Autodesk Fusion 360 part; units mm, degrees
note: some values were not read from the file. Set by a fixed rule: which face or edge a step refers to.
(part 3 of 3)
sketch "Sketch13" plane through (0, 0, 5) normal (0, 0, 1) x (-1, 0, 0)
  line L0 (7, 166) -> (25, 166)
  line L1 (25, 166) -> (25, 167)
  line L2 (25, 167) -> (-35, 167)
  line L3 (-35, 167) -> (-35, 166)
  line L4 (-35, 166) -> (-17, 166)
  line L5 (-17, 166) -> (-17, 164)
  line L6 (-17, 164) -> (-35, 164)
  line L7 (-35, 164) -> (-35, 156)
  line L8 (-35, 156) -> (-17, 156)
  line L9 (-17, 156) -> (-17, 154)
  line L10 (-17, 154) -> (-35, 154)
  line L11 (-35, 154) -> (-35, 146)
  line L12 (-35, 146) -> (-17, 146)
  line L13 (-17, 146) -> (-17, 144)
  line L14 (-17, 144) -> (-35, 144)
  line L15 (-35, 144) -> (-35, 138)
  line L16 (-35, 138) -> (-17, 138)
  line L17 (-17, 138) -> (-17, 136)
  line L18 (-17, 136) -> (-35, 136)
  line L19 (-35, 136) -> (-35, 130)
  line L20 (-35, 130) -> (-17, 130)
  line L21 (-17, 130) -> (-17, 128)
  line L22 (-17, 128) -> (-35, 128)
  line L23 (-35, 128) -> (-35, 122)
  line L24 (-35, 122) -> (-17, 122)
  line L25 (-17, 122) -> (-17, 120)
  line L26 (-17, 120) -> (-35, 120)
  line L27 (-35, 120) -> (-35, 114)
  line L28 (-35, 114) -> (-17, 114)
  line L29 (-17, 114) -> (-17, 112)
  line L30 (-17, 112) -> (-35, 112)
  line L31 (-35, 112) -> (-35, 106)
  line L32 (-35, 106) -> (-17, 106)
  line L33 (-17, 106) -> (-17, 104)
  line L34 (-17, 104) -> (-35, 104)
  line L35 (-35, 104) -> (-35, 98)
  line L36 (-35, 98) -> (-17, 98)
  line L37 (-17, 98) -> (-17, 96)
  line L38 (-17, 96) -> (-35, 96)
  line L39 (-35, 96) -> (-35, 90)
  line L40 (-35, 90) -> (-17, 90)
  line L41 (-17, 90) -> (-17, 88)
  line L42 (-17, 88) -> (-35, 88)
  line L43 (-35, 88) -> (-35, 82)
  line L44 (-35, 82) -> (-17, 82)
  line L45 (-17, 82) -> (-17, 80)
  line L46 (-17, 80) -> (-35, 80)
  line L47 (-35, 80) -> (-35, 74)
  line L48 (-35, 74) -> (-17, 74)
  line L49 (-17, 74) -> (-17, 72)
  line L50 (-17, 72) -> (-35, 72)
  line L51 (-35, 72) -> (-35, 66)
  line L52 (-35, 66) -> (-17, 66)
  line L53 (-17, 66) -> (-17, 64)
  line L54 (-17, 64) -> (-35, 64)
  line L55 (-35, 64) -> (-35, 58)
  line L56 (-35, 58) -> (-17, 58)
  line L57 (-17, 58) -> (-17, 56)
  line L58 (-17, 56) -> (-35, 56)
  line L59 (-35, 56) -> (-35, 50)
  line L60 (-35, 50) -> (-17, 50)
  line L61 (-17, 50) -> (-17, 48)
  line L62 (-17, 48) -> (-35, 48)
  line L63 (-35, 48) -> (-35, 42)
  line L64 (-35, 42) -> (-17, 42)
  line L65 (-17, 42) -> (-17, 40)
  line L66 (-17, 40) -> (-35, 40)
  line L67 (-35, 40) -> (-35, 34)
  line L68 (-35, 34) -> (-17, 34)
  line L69 (-17, 34) -> (-17, 32)
  line L70 (-17, 32) -> (-35, 32)
  line L71 (-35, 32) -> (-35, 26)
  line L72 (-35, 26) -> (-17, 26)
  line L73 (-17, 26) -> (-17, 24)
  line L74 (-17, 24) -> (-35, 24)
  line L75 (-35, 24) -> (-35, 18)
  line L76 (-35, 18) -> (-17, 18)
  line L77 (-17, 18) -> (-17, 16)
  line L78 (-17, 16) -> (-35, 16)
  line L79 (-35, 16) -> (-35, 10)
  line L80 (-35, 10) -> (-17, 10)
  line L81 (-17, 10) -> (-17, 8)
  line L82 (-17, 8) -> (-35, 8)
  line L83 (-35, 8) -> (-35, 2)
  line L84 (-35, 2) -> (-17, 2)
  line L85 (-17, 2) -> (-17, 0)
  line L86 (-17, 0) -> (-35, 0)
  line L87 (-35, 0) -> (-35, -6)
  line L88 (-35, -6) -> (-17, -6)
  line L89 (-17, -6) -> (-17, -8)
  line L90 (-17, -8) -> (-35, -8)
  line L91 (-35, -8) -> (-35, -14)
  line L92 (-35, -14) -> (-17, -14)
  line L93 (-17, -14) -> (-17, -16)
  line L94 (-17, -16) -> (-35, -16)
  line L95 (-35, -16) -> (-35, -22)
  line L96 (-35, -22) -> (-17, -22)
  line L97 (-17, -22) -> (-17, -24)
  line L98 (-17, -24) -> (-35, -24)
  line L99 (-35, -24) -> (-35, -32)
  line L100 (-35, -32) -> (-17, -32)
  line L101 (-17, -32) -> (-17, -34)
  line L102 (-17, -34) -> (-35, -34)
  line L103 (-35, -34) -> (-35, -42)
  line L104 (-35, -42) -> (-40, -42)
  line L105 (-40, -42) -> (-40, -70)
  line L106 (-40, -70) -> (30, -70)
  line L107 (30, -70) -> (30, -42)
  line L108 (30, -42) -> (25, -42)
  line L109 (25, -42) -> (25, -34)
  line L110 (25, -34) -> (7, -34)
  line L111 (7, -34) -> (7, -32)
  line L112 (7, -32) -> (25, -32)
  line L113 (25, -32) -> (25, -24)
  line L114 (25, -24) -> (7, -24)
  line L115 (7, -24) -> (7, -22)
  line L116 (7, -22) -> (25, -22)
  line L117 (25, -22) -> (25, -16)
  line L118 (25, -16) -> (7, -16)
  line L119 (7, -16) -> (7, -14)
  line L120 (7, -14) -> (25, -14)
  line L121 (25, -14) -> (25, -8)
  line L122 (25, -8) -> (7, -8)
  line L123 (7, -8) -> (7, -6)
  line L124 (7, -6) -> (25, -6)
  line L125 (25, -6) -> (25, 0)
  line L126 (25, 0) -> (7, 0)
  line L127 (7, 0) -> (7, 2)
  line L128 (7, 2) -> (25, 2)
  line L129 (25, 2) -> (25, 8)
  line L130 (25, 8) -> (7, 8)
  line L131 (7, 8) -> (7, 10)
  line L132 (7, 10) -> (25, 10)
  line L133 (25, 10) -> (25, 16)
  line L134 (25, 16) -> (7, 16)
  line L135 (7, 16) -> (7, 18)
  line L136 (7, 18) -> (25, 18)
  line L137 (25, 18) -> (25, 24)
  line L138 (25, 24) -> (7, 24)
  line L139 (7, 24) -> (7, 26)
  line L140 (7, 26) -> (25, 26)
  line L141 (25, 26) -> (25, 32)
  line L142 (25, 32) -> (7, 32)
  line L143 (7, 32) -> (7, 34)
  line L144 (7, 34) -> (25, 34)
  line L145 (25, 34) -> (25, 40)
  line L146 (25, 40) -> (7, 40)
  line L147 (7, 40) -> (7, 42)
  line L148 (7, 42) -> (25, 42)
  line L149 (25, 42) -> (25, 48)
  line L150 (25, 48) -> (7, 48)
  line L151 (7, 48) -> (7, 50)
  line L152 (7, 50) -> (25, 50)
  line L153 (25, 50) -> (25, 56)
  line L154 (25, 56) -> (7, 56)
  line L155 (7, 56) -> (7, 58)
  line L156 (7, 58) -> (25, 58)
  line L157 (25, 58) -> (25, 64)
  line L158 (25, 64) -> (7, 64)
  line L159 (7, 64) -> (7, 66)
  line L160 (7, 66) -> (25, 66)
  line L161 (25, 66) -> (25, 72)
  line L162 (25, 72) -> (7, 72)
  line L163 (7, 72) -> (7, 74)
  line L164 (7, 74) -> (25, 74)
  line L165 (25, 74) -> (25, 80)
  line L166 (25, 80) -> (7, 80)
  line L167 (7, 80) -> (7, 82)
  line L168 (7, 82) -> (25, 82)
  line L169 (25, 82) -> (25, 88)
  line L170 (25, 88) -> (7, 88)
  line L171 (7, 88) -> (7, 90)
  line L172 (7, 90) -> (25, 90)
  line L173 (25, 90) -> (25, 96)
  line L174 (25, 96) -> (7, 96)
  line L175 (7, 96) -> (7, 98)
  line L176 (7, 98) -> (25, 98)
  line L177 (25, 98) -> (25, 104)
  line L178 (25, 104) -> (7, 104)
  line L179 (7, 104) -> (7, 106)
  line L180 (7, 106) -> (25, 106)
  line L181 (25, 106) -> (25, 112)
  line L182 (25, 112) -> (7, 112)
  line L183 (7, 112) -> (7, 114)
  line L184 (7, 114) -> (25, 114)
  line L185 (25, 114) -> (25, 120)
  line L186 (25, 120) -> (7, 120)
  line L187 (7, 120) -> (7, 122)
  line L188 (7, 122) -> (25, 122)
  line L189 (25, 122) -> (25, 128)
  line L190 (25, 128) -> (7, 128)
  line L191 (7, 128) -> (7, 130)
  line L192 (7, 130) -> (25, 130)
  line L193 (25, 130) -> (25, 136)
  line L194 (25, 136) -> (7, 136)
  line L195 (7, 136) -> (7, 138)
  line L196 (7, 138) -> (25, 138)
  line L197 (25, 138) -> (25, 144)
  line L198 (25, 144) -> (7, 144)
  line L199 (7, 144) -> (7, 146)
  line L200 (7, 146) -> (25, 146)
  line L201 (25, 146) -> (25, 154)
  line L202 (25, 154) -> (7, 154)
  line L203 (7, 154) -> (7, 156)
  line L204 (7, 156) -> (25, 156)
  line L205 (25, 156) -> (25, 164)
  line L206 (25, 164) -> (7, 164)
  line L207 (7, 164) -> (7, 166)
  line L208 (23, -29) -> (-33, -29)
  line L209 (-33, -29) -> (-33, -27)
  line L210 (-33, -27) -> (23, -27)
  line L211 (23, -27) -> (23, -29)
  line L212 (4, -32) -> (4, -34)
  line L213 (4, -34) -> (-14, -34)
  line L214 (-14, -34) -> (-14, -32)
  line L215 (-14, -32) -> (4, -32)
  line L216 (23, -39) -> (-33, -39)
  line L217 (-33, -39) -> (-33, -37)
  line L218 (-33, -37) -> (23, -37)
  line L219 (23, -37) -> (23, -39)
  line L220 (4, 146) -> (4, 144)
  line L221 (4, 144) -> (-14, 144)
  line L222 (-14, 144) -> (-14, 146)
  line L223 (-14, 146) -> (4, 146)
  line L224 (23, 78) -> (23, 76)
  line L225 (23, 76) -> (-33, 76)
  line L226 (-33, 76) -> (-33, 78)
  line L227 (-33, 78) -> (23, 78)
  line L228 (-33, 94) -> (23, 94)
  line L229 (23, 94) -> (23, 92)
  line L230 (23, 92) -> (-33, 92)
  line L231 (-33, 92) -> (-33, 94)
  line L232 (23, 54) -> (23, 52)
  line L233 (23, 52) -> (-33, 52)
  line L234 (-33, 52) -> (-33, 54)
  line L235 (-33, 54) -> (23, 54)
  line L236 (4, 66) -> (4, 64)
  line L237 (4, 64) -> (-14, 64)
  line L238 (-14, 64) -> (-14, 66)
  line L239 (-14, 66) -> (4, 66)
  line L240 (4, 106) -> (4, 104)
  line L241 (4, 104) -> (-14, 104)
  line L242 (-14, 104) -> (-14, 106)
  line L243 (-14, 106) -> (4, 106)
  line L244 (23, 102) -> (23, 100)
  line L245 (23, 100) -> (-32.9874, 100)
  line L246 (-32.9874, 100) -> (-32.9874, 102)
  line L247 (-32.9874, 102) -> (23, 102)
  line L248 (4, 50) -> (4, 48)
  line L249 (4, 48) -> (-14, 48)
  line L250 (-14, 48) -> (-14, 50)
  line L251 (-14, 50) -> (4, 50)
  line L252 (4, 90) -> (4, 88)
  line L253 (4, 88) -> (-14, 88)
  line L254 (-14, 88) -> (-14, 90)
  line L255 (-14, 90) -> (4, 90)
  line L256 (4, 74) -> (4, 72)
  line L257 (4, 72) -> (-14, 72)
  line L258 (-14, 72) -> (-14, 74)
  line L259 (-14, 74) -> (4, 74)
  line L260 (23, 62) -> (23, 60)
  line L261 (23, 60) -> (-33, 60)
  line L262 (-33, 60) -> (-33, 62)
  line L263 (-33, 62) -> (23, 62)
  line L264 (-33, 116) -> (-33, 118)
  line L265 (-33, 118) -> (23, 118)
  line L266 (23, 118) -> (23, 116)
  line L267 (23, 116) -> (-33, 116)
  line L268 (4, 82) -> (4, 80)
  line L269 (4, 80) -> (-14, 80)
  line L270 (-14, 80) -> (-14, 82)
  line L271 (-14, 82) -> (4, 82)
  line L272 (4, 42) -> (4, 40)
  line L273 (4, 40) -> (-14, 40)
  line L274 (-14, 40) -> (-14, 42)
  line L275 (-14, 42) -> (4, 42)
  line L276 (23, 70) -> (23, 68)
  line L277 (23, 68) -> (-33, 68)
  line L278 (-33, 68) -> (-33, 70)
  line L279 (-33, 70) -> (23, 70)
  line L280 (23, 110) -> (23, 108)
  line L281 (23, 108) -> (-33, 108)
  line L282 (-33, 108) -> (-33, 110)
  line L283 (-33, 110) -> (23, 110)
  line L284 (4, 114) -> (4, 112)
  line L285 (4, 112) -> (-14, 112)
  line L286 (-14, 112) -> (-14, 114)
  line L287 (-14, 114) -> (4, 114)
  line L288 (4, 98) -> (4, 96)
  line L289 (4, 96) -> (-14, 96)
  line L290 (-14, 96) -> (-14, 98)
  line L291 (-14, 98) -> (4, 98)
  line L292 (23, 46.2715) -> (23, 44)
  line L293 (23, 44) -> (-33, 44)
  line L294 (-33, 44) -> (-33, 46.2715)
  line L295 (-33, 46.2715) -> (23, 46.2715)
  line L296 (23, 86) -> (23, 84)
  line L297 (23, 84) -> (-33, 84)
  line L298 (-33, 84) -> (-33, 86)
  line L299 (-33, 86) -> (23, 86)
  line L300 (4, 58) -> (4, 56)
  line L301 (4, 56) -> (-14, 56)
  line L302 (-14, 56) -> (-14, 58)
  line L303 (-14, 58) -> (4, 58)
  line L304 (23, -18) -> (23, -20)
  line L305 (23, -20) -> (-33, -20)
  line L306 (-33, -20) -> (-33, -18)
  line L307 (-33, -18) -> (23, -18)
  line L308 (4, -24) -> (-14, -24)
  line L309 (-14, -24) -> (-14, -22)
  line L310 (-14, -22) -> (4, -22)
  line L311 (4, -22) -> (4, -24)
  line L312 (23, 22) -> (23, 20)
  line L313 (23, 20) -> (-33, 20)
  line L314 (-33, 20) -> (-33, 22)
  line L315 (-33, 22) -> (23, 22)
  line L316 (23, 6) -> (23, 4)
  line L317 (23, 4) -> (-33, 4)
  line L318 (-33, 4) -> (-33, 6)
  line L319 (-33, 6) -> (23, 6)
  line L320 (23, -10) -> (23, -12)
  line L321 (23, -12) -> (-33, -12)
  line L322 (-33, -12) -> (-33, -10)
  line L323 (-33, -10) -> (23, -10)
  line L324 (4, -14) -> (4, -16)
  line L325 (4, -16) -> (-14, -16)
  line L326 (-14, -16) -> (-14, -14)
  line L327 (-14, -14) -> (4, -14)
  line L328 (4, -6) -> (4, -8)
  line L329 (4, -8) -> (-14, -8)
  line L330 (-14, -8) -> (-14, -6)
  line L331 (-14, -6) -> (4, -6)
  line L332 (4, 10) -> (4, 8)
  line L333 (4, 8) -> (-14, 8)
  line L334 (-14, 8) -> (-14, 10)
  line L335 (-14, 10) -> (4, 10)
  line L336 (4, 26) -> (4, 24)
  line L337 (4, 24) -> (-14, 24)
  line L338 (-14, 24) -> (-14, 26)
  line L339 (-14, 26) -> (4, 26)
  line L340 (4, 34) -> (4, 32)
  line L341 (4, 32) -> (-14, 32)
  line L342 (-14, 32) -> (-14, 34)
  line L343 (-14, 34) -> (4, 34)
  line L344 (4, 18) -> (4, 16)
  line L345 (4, 16) -> (-14, 16)
  line L346 (-14, 16) -> (-14, 18)
  line L347 (-14, 18) -> (4, 18)
  line L348 (4, 2) -> (4, 0)
  line L349 (4, 0) -> (-14, 0)
  line L350 (-14, 0) -> (-14, 2)
  line L351 (-14, 2) -> (4, 2)
  line L352 (23, 38) -> (23, 36)
  line L353 (23, 36) -> (-33, 36)
  line L354 (-33, 36) -> (-33, 38)
  line L355 (-33, 38) -> (23, 38)
  line L356 (23, -2) -> (23, -4)
  line L357 (23, -4) -> (-33, -4)
  line L358 (-33, -4) -> (-33, -2)
  line L359 (-33, -2) -> (23, -2)
  line L360 (23, 14) -> (23, 12)
  line L361 (23, 12) -> (-33, 12)
  line L362 (-33, 12) -> (-33, 14)
  line L363 (-33, 14) -> (23, 14)
  line L364 (23, 30) -> (23, 28)
  line L365 (23, 28) -> (-33, 28)
  line L366 (-33, 28) -> (-33, 30)
  line L367 (-33, 30) -> (23, 30)
  line L368 (4, 122) -> (4, 120)
  line L369 (4, 120) -> (-14, 120)
  line L370 (-14, 120) -> (-14, 122)
  line L371 (-14, 122) -> (4, 122)
  line L372 (4, 138) -> (4, 136)
  line L373 (4, 136) -> (-14, 136)
  line L374 (-14, 136) -> (-14, 138)
  line L375 (-14, 138) -> (4, 138)
  line L376 (4, 130) -> (4, 128)
  line L377 (4, 128) -> (-14, 128)
  line L378 (-14, 128) -> (-14, 130)
  line L379 (-14, 130) -> (4, 130)
  line L380 (23, 126) -> (23, 124)
  line L381 (23, 124) -> (-33, 124)
  line L382 (-33, 124) -> (-33, 126)
  line L383 (-33, 126) -> (23, 126)
  line L384 (23, 142) -> (23, 140)
  line L385 (23, 140) -> (-33, 140)
  line L386 (-33, 140) -> (-33, 142)
  line L387 (-33, 142) -> (23, 142)
  line L388 (23, 134) -> (23, 132)
  line L389 (23, 132) -> (-33, 132)
  line L390 (-33, 132) -> (-33, 134)
  line L391 (-33, 134) -> (23, 134)
  line L392 (23, 151) -> (23, 149)
  line L393 (23, 149) -> (-33, 149)
  line L394 (-33, 149) -> (-33, 151)
  line L395 (-33, 151) -> (23, 151)
  line L396 (4, 156) -> (4, 154)
  line L397 (4, 154) -> (-14, 154)
  line L398 (-14, 154) -> (-14, 156)
  line L399 (-14, 156) -> (4, 156)
  line L400 (23, 161) -> (23, 159)
  line L401 (23, 159) -> (-33, 159)
  line L402 (-33, 159) -> (-33, 161)
  line L403 (-33, 161) -> (23, 161)
  line L404 (-14, 164) -> (-14, 166)
  line L405 (-14, 166) -> (4, 166)
  line L406 (4, 166) -> (4, 164)
  line L407 (4, 164) -> (-14, 164)
  line L408 (30, -42) -> (-40, -42)
  line L409 (-40, -42) -> (-40, -70)
  line L410 (-40, -70) -> (30, -70)
  line L411 (30, -70) -> (30, -42)
  constraint horizontal L408
  constraint vertical L409
  constraint horizontal L410
  constraint vertical L411
  constraint coincident L105.end L106.start
  constraint coincident L107.end L108.start
extrude "Extrude20" add sketch "Sketch13" along normal blind 2.5 contours L104 L105 L106 L107 L108 L408 L409 L410 L411
sketch "Sketch14" plane through (0, 0, 0) normal (0, 0, -1) x (1, 0, 0)
  line L0 (-25, 166) -> (-7, 166)
  line L1 (-7, 166) -> (-7, 164)
  line L2 (-7, 164) -> (-25, 164)
  line L3 (-25, 164) -> (-25, 156)
  line L4 (-25, 156) -> (-7, 156)
  line L5 (-7, 156) -> (-7, 154)
  line L6 (-7, 154) -> (-25, 154)
  line L7 (-25, 154) -> (-25, 146)
  line L8 (-25, 146) -> (-7, 146)
  line L9 (-7, 146) -> (-7, 144)
  line L10 (-7, 144) -> (-25, 144)
  line L11 (-25, 144) -> (-25, 138)
  line L12 (-25, 138) -> (-7, 138)
  line L13 (-7, 138) -> (-7, 136)
  line L14 (-7, 136) -> (-25, 136)
  line L15 (-25, 136) -> (-25, 130)
  line L16 (-25, 130) -> (-7, 130)
  line L17 (-7, 130) -> (-7, 128)
  line L18 (-7, 128) -> (-25, 128)
  line L19 (-25, 128) -> (-25, 122)
  line L20 (-25, 122) -> (-7, 122)
  line L21 (-7, 122) -> (-7, 120)
  line L22 (-7, 120) -> (-25, 120)
  line L23 (-25, 120) -> (-25, 114)
  line L24 (-25, 114) -> (-7, 114)
  line L25 (-7, 114) -> (-7, 112)
  line L26 (-7, 112) -> (-25, 112)
  line L27 (-25, 112) -> (-25, 106)
  line L28 (-25, 106) -> (-7, 106)
  line L29 (-7, 106) -> (-7, 104)
  line L30 (-7, 104) -> (-25, 104)
  line L31 (-25, 104) -> (-25, 98)
  line L32 (-25, 98) -> (-7, 98)
  line L33 (-7, 98) -> (-7, 96)
  line L34 (-7, 96) -> (-25, 96)
  line L35 (-25, 96) -> (-25, 90)
  line L36 (-25, 90) -> (-7, 90)
  line L37 (-7, 90) -> (-7, 88)
  line L38 (-7, 88) -> (-25, 88)
  line L39 (-25, 88) -> (-25, 82)
  line L40 (-25, 82) -> (-7, 82)
  line L41 (-7, 82) -> (-7, 80)
  line L42 (-7, 80) -> (-25, 80)
  line L43 (-25, 80) -> (-25, 74)
  line L44 (-25, 74) -> (-7, 74)
  line L45 (-7, 74) -> (-7, 72)
  line L46 (-7, 72) -> (-25, 72)
  line L47 (-25, 72) -> (-25, 66)
  line L48 (-25, 66) -> (-7, 66)
  line L49 (-7, 66) -> (-7, 64)
  line L50 (-7, 64) -> (-25, 64)
  line L51 (-25, 64) -> (-25, 58)
  line L52 (-25, 58) -> (-7, 58)
  line L53 (-7, 58) -> (-7, 56)
  line L54 (-7, 56) -> (-25, 56)
  line L55 (-25, 56) -> (-25, 50)
  line L56 (-25, 50) -> (-7, 50)
  line L57 (-7, 50) -> (-7, 48)
  line L58 (-7, 48) -> (-25, 48)
  line L59 (-25, 48) -> (-25, 42)
  line L60 (-25, 42) -> (-7, 42)
  line L61 (-7, 42) -> (-7, 40)
  line L62 (-7, 40) -> (-25, 40)
  line L63 (-25, 40) -> (-25, 34)
  line L64 (-25, 34) -> (-7, 34)
  line L65 (-7, 34) -> (-7, 32)
  line L66 (-7, 32) -> (-25, 32)
  line L67 (-25, 32) -> (-25, 26)
  line L68 (-25, 26) -> (-7, 26)
  line L69 (-7, 26) -> (-7, 24)
  line L70 (-7, 24) -> (-25, 24)
  line L71 (-25, 24) -> (-25, 18)
  line L72 (-25, 18) -> (-7, 18)
  line L73 (-7, 18) -> (-7, 16)
  line L74 (-7, 16) -> (-25, 16)
  line L75 (-25, 16) -> (-25, 10)
  line L76 (-25, 10) -> (-7, 10)
  line L77 (-7, 10) -> (-7, 8)
  line L78 (-7, 8) -> (-25, 8)
  line L79 (-25, 8) -> (-25, 2)
  line L80 (-25, 2) -> (-7, 2)
  line L81 (-7, 2) -> (-7, 0)
  line L82 (-7, 0) -> (-25, 0)
  line L83 (-25, 0) -> (-25, -6)
  line L84 (-25, -6) -> (-7, -6)
  line L85 (-7, -6) -> (-7, -8)
  line L86 (-7, -8) -> (-25, -8)
  line L87 (-25, -8) -> (-25, -14)
  line L88 (-25, -14) -> (-7, -14)
  line L89 (-7, -14) -> (-7, -16)
  line L90 (-7, -16) -> (-25, -16)
  line L91 (-25, -16) -> (-25, -22)
  line L92 (-25, -22) -> (-7, -22)
  line L93 (-7, -22) -> (-7, -24)
  line L94 (-7, -24) -> (-25, -24)
  line L95 (-25, -24) -> (-25, -32)
  line L96 (-25, -32) -> (-7, -32)
  line L97 (-7, -32) -> (-7, -34)
  line L98 (-7, -34) -> (-25, -34)
  line L99 (-25, -34) -> (-25, -42)
  line L100 (-25, -42) -> (-30, -42)
  line L101 (-30, -42) -> (-30, -70)
  line L102 (-30, -70) -> (40, -70)
  line L103 (40, -70) -> (40, -42)
  line L104 (40, -42) -> (35, -42)
  line L105 (35, -42) -> (35, -34)
  line L106 (35, -34) -> (17, -34)
  line L107 (17, -34) -> (17, -32)
  line L108 (17, -32) -> (35, -32)
  line L109 (35, -32) -> (35, -24)
  line L110 (35, -24) -> (17, -24)
  line L111 (17, -24) -> (17, -22)
  line L112 (17, -22) -> (35, -22)
  line L113 (35, -22) -> (35, -16)
  line L114 (35, -16) -> (17, -16)
  line L115 (17, -16) -> (17, -14)
  line L116 (17, -14) -> (35, -14)
  line L117 (35, -14) -> (35, -8)
  line L118 (35, -8) -> (17, -8)
  line L119 (17, -8) -> (17, -6)
  line L120 (17, -6) -> (35, -6)
  line L121 (35, -6) -> (35, 0)
  line L122 (35, 0) -> (17, 0)
  line L123 (17, 0) -> (17, 2)
  line L124 (17, 2) -> (35, 2)
  line L125 (35, 2) -> (35, 8)
  line L126 (35, 8) -> (17, 8)
  line L127 (17, 8) -> (17, 10)
  line L128 (17, 10) -> (35, 10)
  line L129 (35, 10) -> (35, 16)
  line L130 (35, 16) -> (17, 16)
  line L131 (17, 16) -> (17, 18)
  line L132 (17, 18) -> (35, 18)
  line L133 (35, 18) -> (35, 24)
  line L134 (35, 24) -> (17, 24)
  line L135 (17, 24) -> (17, 26)
  line L136 (17, 26) -> (35, 26)
  line L137 (35, 26) -> (35, 32)
  line L138 (35, 32) -> (17, 32)
  line L139 (17, 32) -> (17, 34)
  line L140 (17, 34) -> (35, 34)
  line L141 (35, 34) -> (35, 40)
  line L142 (35, 40) -> (17, 40)
  line L143 (17, 40) -> (17, 42)
  line L144 (17, 42) -> (35, 42)
  line L145 (35, 42) -> (35, 48)
  line L146 (35, 48) -> (17, 48)
  line L147 (17, 48) -> (17, 50)
  line L148 (17, 50) -> (35, 50)
  line L149 (35, 50) -> (35, 56)
  line L150 (35, 56) -> (17, 56)
  line L151 (17, 56) -> (17, 58)
  line L152 (17, 58) -> (35, 58)
  line L153 (35, 58) -> (35, 64)
  line L154 (35, 64) -> (17, 64)
  line L155 (17, 64) -> (17, 66)
  line L156 (17, 66) -> (35, 66)
  line L157 (35, 66) -> (35, 72)
  line L158 (35, 72) -> (17, 72)
  line L159 (17, 72) -> (17, 74)
  line L160 (17, 74) -> (35, 74)
  line L161 (35, 74) -> (35, 80)
  line L162 (35, 80) -> (17, 80)
  line L163 (17, 80) -> (17, 82)
  line L164 (17, 82) -> (35, 82)
  line L165 (35, 82) -> (35, 88)
  line L166 (35, 88) -> (17, 88)
  line L167 (17, 88) -> (17, 90)
  line L168 (17, 90) -> (35, 90)
  line L169 (35, 90) -> (35, 96)
  line L170 (35, 96) -> (17, 96)
  line L171 (17, 96) -> (17, 98)
  line L172 (17, 98) -> (35, 98)
  line L173 (35, 98) -> (35, 104)
  line L174 (35, 104) -> (17, 104)
  line L175 (17, 104) -> (17, 106)
  line L176 (17, 106) -> (35, 106)
  line L177 (35, 106) -> (35, 112)
  line L178 (35, 112) -> (17, 112)
  line L179 (17, 112) -> (17, 114)
  line L180 (17, 114) -> (35, 114)
  line L181 (35, 114) -> (35, 120)
  line L182 (35, 120) -> (17, 120)
  line L183 (17, 120) -> (17, 122)
  line L184 (17, 122) -> (35, 122)
  line L185 (35, 122) -> (35, 128)
  line L186 (35, 128) -> (17, 128)
  line L187 (17, 128) -> (17, 130)
  line L188 (17, 130) -> (35, 130)
  line L189 (35, 130) -> (35, 136)
  line L190 (35, 136) -> (17, 136)
  line L191 (17, 136) -> (17, 138)
  line L192 (17, 138) -> (35, 138)
  line L193 (35, 138) -> (35, 144)
  line L194 (35, 144) -> (17, 144)
  line L195 (17, 144) -> (17, 146)
  line L196 (17, 146) -> (35, 146)
  line L197 (35, 146) -> (35, 154)
  line L198 (35, 154) -> (17, 154)
  line L199 (17, 154) -> (17, 156)
  line L200 (17, 156) -> (35, 156)
  line L201 (35, 156) -> (35, 164)
  line L202 (35, 164) -> (17, 164)
  line L203 (17, 164) -> (17, 166)
  line L204 (17, 166) -> (35, 166)
  line L205 (35, 166) -> (35, 167)
  line L206 (35, 167) -> (-25, 167)
  line L207 (-25, 167) -> (-25, 166)
  line L208 (33, -29) -> (-23, -29)
  line L209 (-23, -29) -> (-23, -27)
  line L210 (-23, -27) -> (33, -27)
  line L211 (33, -27) -> (33, -29)
  line L212 (-4, -34) -> (-4, -32)
  line L213 (-4, -32) -> (14, -32)
  line L214 (14, -32) -> (14, -34)
  line L215 (14, -34) -> (-4, -34)
  line L216 (33, -39) -> (-23, -39)
  line L217 (-23, -39) -> (-23, -37)
  line L218 (-23, -37) -> (33, -37)
  line L219 (33, -37) -> (33, -39)
  line L220 (-4, 144) -> (-4, 146)
  line L221 (-4, 146) -> (14, 146)
  line L222 (14, 146) -> (14, 144)
  line L223 (14, 144) -> (-4, 144)
  line L224 (-23, 76) -> (-23, 78)
  line L225 (-23, 78) -> (33, 78)
  line L226 (33, 78) -> (33, 76)
  line L227 (33, 76) -> (-23, 76)
  line L228 (-23, 94) -> (33, 94)
  line L229 (33, 94) -> (33, 92)
  line L230 (33, 92) -> (-23, 92)
  line L231 (-23, 92) -> (-23, 94)
  line L232 (-23, 52) -> (-23, 54)
  line L233 (-23, 54) -> (33, 54)
  line L234 (33, 54) -> (33, 52)
  line L235 (33, 52) -> (-23, 52)
  line L236 (-4, 64) -> (-4, 66)
  line L237 (-4, 66) -> (14, 66)
  line L238 (14, 66) -> (14, 64)
  line L239 (14, 64) -> (-4, 64)
  line L240 (-4, 104) -> (-4, 106)
  line L241 (-4, 106) -> (14, 106)
  line L242 (14, 106) -> (14, 104)
  line L243 (14, 104) -> (-4, 104)
  line L244 (-23, 100) -> (-23, 102)
  line L245 (-23, 102) -> (32.9874, 102)
  line L246 (32.9874, 102) -> (32.9874, 100)
  line L247 (32.9874, 100) -> (-23, 100)
  line L248 (-4, 48) -> (-4, 50)
  line L249 (-4, 50) -> (14, 50)
  line L250 (14, 50) -> (14, 48)
  line L251 (14, 48) -> (-4, 48)
  line L252 (-4, 88) -> (-4, 90)
  line L253 (-4, 90) -> (14, 90)
  line L254 (14, 90) -> (14, 88)
  line L255 (14, 88) -> (-4, 88)
  line L256 (-4, 72) -> (-4, 74)
  line L257 (-4, 74) -> (14, 74)
  line L258 (14, 74) -> (14, 72)
  line L259 (14, 72) -> (-4, 72)
  line L260 (-23, 60) -> (-23, 62)
  line L261 (-23, 62) -> (33, 62)
  line L262 (33, 62) -> (33, 60)
  line L263 (33, 60) -> (-23, 60)
  line L264 (33, 118) -> (33, 116)
  line L265 (33, 116) -> (-23, 116)
  line L266 (-23, 116) -> (-23, 118)
  line L267 (-23, 118) -> (33, 118)
  line L268 (-4, 80) -> (-4, 82)
  line L269 (-4, 82) -> (14, 82)
  line L270 (14, 82) -> (14, 80)
  line L271 (14, 80) -> (-4, 80)
  line L272 (-4, 40) -> (-4, 42)
  line L273 (-4, 42) -> (14, 42)
  line L274 (14, 42) -> (14, 40)
  line L275 (14, 40) -> (-4, 40)
  line L276 (-23, 68) -> (-23, 70)
  line L277 (-23, 70) -> (33, 70)
  line L278 (33, 70) -> (33, 68)
  line L279 (33, 68) -> (-23, 68)
  line L280 (-23, 108) -> (-23, 110)
  line L281 (-23, 110) -> (33, 110)
  line L282 (33, 110) -> (33, 108)
  line L283 (33, 108) -> (-23, 108)
  line L284 (-4, 112) -> (-4, 114)
  line L285 (-4, 114) -> (14, 114)
  line L286 (14, 114) -> (14, 112)
  line L287 (14, 112) -> (-4, 112)
  line L288 (-4, 96) -> (-4, 98)
  line L289 (-4, 98) -> (14, 98)
  line L290 (14, 98) -> (14, 96)
  line L291 (14, 96) -> (-4, 96)
  line L292 (-23, 44) -> (-23, 46.2715)
  line L293 (-23, 46.2715) -> (33, 46.2715)
  line L294 (33, 46.2715) -> (33, 44)
  line L295 (33, 44) -> (-23, 44)
  line L296 (-23, 84) -> (-23, 86)
  line L297 (-23, 86) -> (33, 86)
  line L298 (33, 86) -> (33, 84)
  line L299 (33, 84) -> (-23, 84)
  line L300 (-4, 56) -> (-4, 58)
  line L301 (-4, 58) -> (14, 58)
  line L302 (14, 58) -> (14, 56)
  line L303 (14, 56) -> (-4, 56)
  line L304 (14, -24) -> (-4, -24)
  line L305 (-4, -24) -> (-4, -22)
  line L306 (-4, -22) -> (14, -22)
  line L307 (14, -22) -> (14, -24)
  line L308 (-23, -20) -> (-23, -18)
  line L309 (-23, -18) -> (33, -18)
  line L310 (33, -18) -> (33, -20)
  line L311 (33, -20) -> (-23, -20)
  line L312 (-23, 20) -> (-23, 22)
  line L313 (-23, 22) -> (33, 22)
  line L314 (33, 22) -> (33, 20)
  line L315 (33, 20) -> (-23, 20)
  line L316 (-23, 4) -> (-23, 6)
  line L317 (-23, 6) -> (33, 6)
  line L318 (33, 6) -> (33, 4)
  line L319 (33, 4) -> (-23, 4)
  line L320 (-23, -12) -> (-23, -10)
  line L321 (-23, -10) -> (33, -10)
  line L322 (33, -10) -> (33, -12)
  line L323 (33, -12) -> (-23, -12)
  line L324 (-4, -16) -> (-4, -14)
  line L325 (-4, -14) -> (14, -14)
  line L326 (14, -14) -> (14, -16)
  line L327 (14, -16) -> (-4, -16)
  line L328 (-4, -8) -> (-4, -6)
  line L329 (-4, -6) -> (14, -6)
  line L330 (14, -6) -> (14, -8)
  line L331 (14, -8) -> (-4, -8)
  line L332 (-4, 8) -> (-4, 10)
  line L333 (-4, 10) -> (14, 10)
  line L334 (14, 10) -> (14, 8)
  line L335 (14, 8) -> (-4, 8)
  line L336 (-4, 24) -> (-4, 26)
  line L337 (-4, 26) -> (14, 26)
  line L338 (14, 26) -> (14, 24)
  line L339 (14, 24) -> (-4, 24)
  line L340 (-4, 32) -> (-4, 34)
  line L341 (-4, 34) -> (14, 34)
  line L342 (14, 34) -> (14, 32)
  line L343 (14, 32) -> (-4, 32)
  line L344 (-4, 16) -> (-4, 18)
  line L345 (-4, 18) -> (14, 18)
  line L346 (14, 18) -> (14, 16)
  line L347 (14, 16) -> (-4, 16)
  line L348 (-4, 0) -> (-4, 2)
  line L349 (-4, 2) -> (14, 2)
  line L350 (14, 2) -> (14, 0)
  line L351 (14, 0) -> (-4, 0)
  line L352 (-23, 36) -> (-23, 38)
  line L353 (-23, 38) -> (33, 38)
  line L354 (33, 38) -> (33, 36)
  line L355 (33, 36) -> (-23, 36)
  line L356 (-23, -4) -> (-23, -2)
  line L357 (-23, -2) -> (33, -2)
  line L358 (33, -2) -> (33, -4)
  line L359 (33, -4) -> (-23, -4)
  line L360 (-23, 12) -> (-23, 14)
  line L361 (-23, 14) -> (33, 14)
  line L362 (33, 14) -> (33, 12)
  line L363 (33, 12) -> (-23, 12)
  line L364 (-23, 28) -> (-23, 30)
  line L365 (-23, 30) -> (33, 30)
  line L366 (33, 30) -> (33, 28)
  line L367 (33, 28) -> (-23, 28)
  line L368 (-4, 120) -> (-4, 122)
  line L369 (-4, 122) -> (14, 122)
  line L370 (14, 122) -> (14, 120)
  line L371 (14, 120) -> (-4, 120)
  line L372 (-4, 136) -> (-4, 138)
  line L373 (-4, 138) -> (14, 138)
  line L374 (14, 138) -> (14, 136)
  line L375 (14, 136) -> (-4, 136)
  line L376 (-4, 128) -> (-4, 130)
  line L377 (-4, 130) -> (14, 130)
  line L378 (14, 130) -> (14, 128)
  line L379 (14, 128) -> (-4, 128)
  line L380 (-23, 124) -> (-23, 126)
  line L381 (-23, 126) -> (33, 126)
  line L382 (33, 126) -> (33, 124)
  line L383 (33, 124) -> (-23, 124)
  line L384 (-23, 140) -> (-23, 142)
  line L385 (-23, 142) -> (33, 142)
  line L386 (33, 142) -> (33, 140)
  line L387 (33, 140) -> (-23, 140)
  line L388 (-23, 132) -> (-23, 134)
  line L389 (-23, 134) -> (33, 134)
  line L390 (33, 134) -> (33, 132)
  line L391 (33, 132) -> (-23, 132)
  line L392 (-23, 149) -> (-23, 151)
  line L393 (-23, 151) -> (33, 151)
  line L394 (33, 151) -> (33, 149)
  line L395 (33, 149) -> (-23, 149)
  line L396 (-4, 154) -> (-4, 156)
  line L397 (-4, 156) -> (14, 156)
  line L398 (14, 156) -> (14, 154)
  line L399 (14, 154) -> (-4, 154)
  line L400 (-23, 159) -> (-23, 161)
  line L401 (-23, 161) -> (33, 161)
  line L402 (33, 161) -> (33, 159)
  line L403 (33, 159) -> (-23, 159)
  line L404 (14, 166) -> (14, 164)
  line L405 (14, 164) -> (-4, 164)
  line L406 (-4, 164) -> (-4, 166)
  line L407 (-4, 166) -> (14, 166)
  line L408 (40, -70) -> (-30, -70)
  line L409 (-30, -70) -> (-30, -42)
  line L410 (-30, -42) -> (40, -42)
  line L411 (40, -42) -> (40, -70)
  constraint horizontal L408
  constraint vertical L409
  constraint horizontal L410
  constraint vertical L411
  constraint coincident L100.end L101.start
  constraint coincident L102.end L103.start
extrude "Extrude21" add sketch "Sketch14" along normal blind 2.5 contours L100 L101 L102 L103 L104 L408 L409 L410 L411
sketch "Sketch16" plane through (0, 0, -2.5) normal (0, 0, -1) x (1, 0, 0)
  line L0 (40, -42) -> (-30, -42)
  line L1 (-30, -42) -> (-30, -70)
  line L2 (-30, -70) -> (40, -70)
  line L3 (40, -70) -> (40, -42)
  line L4 (-30, -60) -> (-25, -60)
  line L5 (40, -60) -> (35, -60)
  line L6 (0, -42) -> (0, -52)
  line L7 (0, -70) -> (0, -60)
  line L8 (-25, -60) -> (35, -60)
  line L9 (35, -60) -> (35, -52)
  line L10 (35, -52) -> (-25, -52)
  line L11 (-25, -52) -> (-25, -60)
  dimension "d147" = 5
  dimension "d148" = 10
  dimension "d149" = 10
  constraint coincident L1 L4.start
  constraint perpendicular L1 L4
  constraint coincident L3 L5.start
  constraint perpendicular L3 L5
  constraint coincident L2 L7.start
  constraint perpendicular L2 L7
  constraint horizontal L8
  constraint vertical L9
  constraint horizontal L10
  constraint vertical L11
  measures "d147" distance of L4.start L4.end
  measures "d148" distance of L6.start L6.end
  measures "d149" distance of L7.start L7.end
extrude "Extrude22" cut sketch "Sketch16" against normal blind 10 contours L8 L9 L10 L11
extrude "Extrude23" cut 1 faces at (-5, 66.6667, -2.5) along direction (0, 0, 1) blind 2
extrude "Extrude24" cut 1 faces at (-5, 66.6667, -0.5) along direction (0, 0, 1) blind 0.5
extrude "Extrude25" add 1 faces at (-5, 60, 2.5) along direction (0, -1, 0) blind 8
extrude "Extrude26" add 1 faces at (-5, 60.6667, 7.5) along direction (0, 0, 1) blind 2.5
sketch "Sketch17" plane through (35, 0, 0) normal (1, 0, 0) x (0, 1, 0)
  line L0 (6, 0) -> (6, 5)
  line L1 (6, 5) -> (0, 5)
  line L2 (0, 5) -> (0, 0)
  line L3 (0, 0) -> (6, 0)
sketch "Sketch18" plane through (40, 0, 0) normal (1, 0, 0) x (0, 1, 0)
  line L0 (42, 0) -> (70, 0)
  line L1 (70, 0) -> (70, 10)
  line L2 (70, 10) -> (42, 10)
  line L3 (42, 10) -> (42, 0)
  line L4 (43.5, 7.5) -> (68.5, 7.5)
  line L5 (68.5, 7.5) -> (68.5, 1.5)
  line L6 (68.5, 1.5) -> (43.5, 1.5)
  line L7 (43.5, 1.5) -> (43.5, 7.5)
  dimension "d160" = 25
  dimension "d161" = 6
  constraint perpendicular L4 L5
  constraint parallel L4 L6
  constraint parallel L5 L7
  constraint parallel L0 L4
  measures "d160" distance of L4.start L4.end
  measures "d161" distance of L4.start L6.end
extrude "Extrude27" cut sketch "Sketch18" against normal blind 10 contours L4 L5 L6 L7
extrude "Extrude28" cut 1 faces at (30, 51.8333, 5.5) along direction (-1, 0, 0) blind 120
extrude "Extrude29" add 1 faces at (-5, 60.6667, 10) along direction (0, 0, 1) blind 1.5
extrude "Extrude30" add 1 faces at (-6.6667, 52.1667, 1.5) along direction (0, 0, 1) blind 2.5
extrude "Extrude31" add 1 faces at (16.6667, 43.5, 5.8333) along direction (0, 1, 0) blind 7
extrude "Extrude32" add 1 faces at (16.6667, 70, 9.3333) along direction (0, 1, 0) blind 10
extrude "Extrude33" cut 1 faces at (16.6667, 68.5, 6.6667) along direction (0, 1, 0) blind 5
move_face "OffsetFaces1" offset -0.5 1 faces at (-6.6667, 64.1667, 4)
extrude "Extrude34" cut 1 faces at (16.6667, 63, 7.5) along direction (0, 0, 1) blind 3
extrude "Extrude35" add 1 faces at (-5, 60.6667, 11.5) along direction (0, 0, 1) blind 4
extrude "Extrude36" cut 1 faces at (16.6667, 63, 10.5) along direction (0, 0, 1) blind 1
extrude "Extrude37" add 1 faces at (16.6667, 63, 11.5) along direction (0, 0, -1) blind 1
extrude "Extrude38" add 1 faces at (-6.6667, 64.1667, 3.5) along direction (0, 0, 1) blind 1
extrude "Extrude39" cut 1 faces at (16.6667, 50.5, 5.6667) along direction (0, -1, 0) blind 1.5
fillet "Fillet3" radius 4 1 edges at (5, 42, 5)
extrude "Extrude40" cut 1 faces at (15, -167, 1.6667) along direction (0, 1, 0) blind 3
sketch "Sketch19" plane through (0, 0, 5) normal (0, 0, 1) x (-1, 0, 0)
  line L0 (25, 164) -> (-35, 164)
  line L1 (-35, 164) -> (-35, 156)
  line L2 (-35, 156) -> (-17, 156)
  line L3 (-17, 156) -> (-17, 154)
  line L4 (-17, 154) -> (-35, 154)
  line L5 (-35, 154) -> (-35, 146)
  line L6 (-35, 146) -> (-17, 146)
  line L7 (-17, 146) -> (-17, 144)
  line L8 (-17, 144) -> (-35, 144)
  line L9 (-35, 144) -> (-35, 138)
  line L10 (-35, 138) -> (-17, 138)
  line L11 (-17, 138) -> (-17, 136)
  line L12 (-17, 136) -> (-35, 136)
  line L13 (-35, 136) -> (-35, 130)
  line L14 (-35, 130) -> (-17, 130)
  line L15 (-17, 130) -> (-17, 128)
  line L16 (-17, 128) -> (-35, 128)
  line L17 (-35, 128) -> (-35, 122)
  line L18 (-35, 122) -> (-17, 122)
  line L19 (-17, 122) -> (-17, 120)
  line L20 (-17, 120) -> (-35, 120)
  line L21 (-35, 120) -> (-35, 114)
  line L22 (-35, 114) -> (-17, 114)
  line L23 (-17, 114) -> (-17, 112)
  line L24 (-17, 112) -> (-35, 112)
  line L25 (-35, 112) -> (-35, 106)
  line L26 (-35, 106) -> (-17, 106)
  line L27 (-17, 106) -> (-17, 104)
  line L28 (-17, 104) -> (-35, 104)
  line L29 (-35, 104) -> (-35, 98)
  line L30 (-35, 98) -> (-17, 98)
  line L31 (-17, 98) -> (-17, 96)
  line L32 (-17, 96) -> (-35, 96)
  line L33 (-35, 96) -> (-35, 90)
  line L34 (-35, 90) -> (-17, 90)
  line L35 (-17, 90) -> (-17, 88)
  line L36 (-17, 88) -> (-35, 88)
  line L37 (-35, 88) -> (-35, 82)
  line L38 (-35, 82) -> (-17, 82)
  line L39 (-17, 82) -> (-17, 80)
  line L40 (-17, 80) -> (-35, 80)
  line L41 (-35, 80) -> (-35, 74)
  line L42 (-35, 74) -> (-17, 74)
  line L43 (-17, 74) -> (-17, 72)
  line L44 (-17, 72) -> (-35, 72)
  line L45 (-35, 72) -> (-35, 66)
  line L46 (-35, 66) -> (-17, 66)
  line L47 (-17, 66) -> (-17, 64)
  line L48 (-17, 64) -> (-35, 64)
  line L49 (-35, 64) -> (-35, 58)
  line L50 (-35, 58) -> (-17, 58)
  line L51 (-17, 58) -> (-17, 56)
  line L52 (-17, 56) -> (-35, 56)
  line L53 (-35, 56) -> (-35, 50)
  line L54 (-35, 50) -> (-17, 50)
  line L55 (-17, 50) -> (-17, 48)
  line L56 (-17, 48) -> (-35, 48)
  line L57 (-35, 48) -> (-35, 42)
  line L58 (-35, 42) -> (-17, 42)
  line L59 (-17, 42) -> (-17, 40)
  line L60 (-17, 40) -> (-35, 40)
  line L61 (-35, 40) -> (-35, 34)
  line L62 (-35, 34) -> (-17, 34)
  line L63 (-17, 34) -> (-17, 32)
  line L64 (-17, 32) -> (-35, 32)
  line L65 (-35, 32) -> (-35, 26)
  line L66 (-35, 26) -> (-17, 26)
  line L67 (-17, 26) -> (-17, 24)
  line L68 (-17, 24) -> (-35, 24)
  line L69 (-35, 24) -> (-35, 18)
  line L70 (-35, 18) -> (-17, 18)
  line L71 (-17, 18) -> (-17, 16)
  line L72 (-17, 16) -> (-35, 16)
  line L73 (-35, 16) -> (-35, 10)
  line L74 (-35, 10) -> (-17, 10)
  line L75 (-17, 10) -> (-17, 8)
  line L76 (-17, 8) -> (-35, 8)
  line L77 (-35, 8) -> (-35, 2)
  line L78 (-35, 2) -> (-17, 2)
  line L79 (-17, 2) -> (-17, 0)
  line L80 (-17, 0) -> (-35, 0)
  line L81 (-35, 0) -> (-35, -6)
  line L82 (-35, -6) -> (-17, -6)
  line L83 (-17, -6) -> (-17, -8)
  line L84 (-17, -8) -> (-35, -8)
  line L85 (-35, -8) -> (-35, -14)
  line L86 (-35, -14) -> (-17, -14)
  line L87 (-17, -14) -> (-17, -16)
  line L88 (-17, -16) -> (-35, -16)
  line L89 (-35, -16) -> (-35, -22)
  line L90 (-35, -22) -> (-17, -22)
  line L91 (-17, -22) -> (-17, -24)
  line L92 (-17, -24) -> (-35, -24)
  line L93 (-35, -24) -> (-35, -32)
  line L94 (-35, -32) -> (-17, -32)
  line L95 (-17, -32) -> (-17, -34)
  line L96 (-17, -34) -> (-35, -34)
  line L97 (-35, -34) -> (-35, -38)
  line L98 (-35, -38) -> (-33, -38)
  line L99 (-33, -38) -> (-33, -37)
  line L100 (-33, -37) -> (23, -37)
  line L101 (23, -37) -> (23, -38)
  line L102 (23, -38) -> (25, -38)
  line L103 (25, -38) -> (25, -34)
  line L104 (25, -34) -> (7, -34)
  line L105 (7, -34) -> (7, -32)
  line L106 (7, -32) -> (25, -32)
  line L107 (25, -32) -> (25, -24)
  line L108 (25, -24) -> (7, -24)
  line L109 (7, -24) -> (7, -22)
  line L110 (7, -22) -> (25, -22)
  line L111 (25, -22) -> (25, -16)
  line L112 (25, -16) -> (7, -16)
  line L113 (7, -16) -> (7, -14)
  line L114 (7, -14) -> (25, -14)
  line L115 (25, -14) -> (25, -8)
  line L116 (25, -8) -> (7, -8)
  line L117 (7, -8) -> (7, -6)
  line L118 (7, -6) -> (25, -6)
  line L119 (25, -6) -> (25, 0)
  line L120 (25, 0) -> (7, 0)
  line L121 (7, 0) -> (7, 2)
  line L122 (7, 2) -> (25, 2)
  line L123 (25, 2) -> (25, 8)
  line L124 (25, 8) -> (7, 8)
  line L125 (7, 8) -> (7, 10)
  line L126 (7, 10) -> (25, 10)
  line L127 (25, 10) -> (25, 16)
  line L128 (25, 16) -> (7, 16)
  line L129 (7, 16) -> (7, 18)
  line L130 (7, 18) -> (25, 18)
  line L131 (25, 18) -> (25, 24)
  line L132 (25, 24) -> (7, 24)
  line L133 (7, 24) -> (7, 26)
  line L134 (7, 26) -> (25, 26)
  line L135 (25, 26) -> (25, 32)
  line L136 (25, 32) -> (7, 32)
  line L137 (7, 32) -> (7, 34)
  line L138 (7, 34) -> (25, 34)
  line L139 (25, 34) -> (25, 40)
  line L140 (25, 40) -> (7, 40)
  line L141 (7, 40) -> (7, 42)
  line L142 (7, 42) -> (25, 42)
  line L143 (25, 42) -> (25, 48)
  line L144 (25, 48) -> (7, 48)
  line L145 (7, 48) -> (7, 50)
  line L146 (7, 50) -> (25, 50)
  line L147 (25, 50) -> (25, 56)
  line L148 (25, 56) -> (7, 56)
  line L149 (7, 56) -> (7, 58)
  line L150 (7, 58) -> (25, 58)
  line L151 (25, 58) -> (25, 64)
  line L152 (25, 64) -> (7, 64)
  line L153 (7, 64) -> (7, 66)
  line L154 (7, 66) -> (25, 66)
  line L155 (25, 66) -> (25, 72)
  line L156 (25, 72) -> (7, 72)
  line L157 (7, 72) -> (7, 74)
  line L158 (7, 74) -> (25, 74)
  line L159 (25, 74) -> (25, 80)
  line L160 (25, 80) -> (7, 80)
  line L161 (7, 80) -> (7, 82)
  line L162 (7, 82) -> (25, 82)
  line L163 (25, 82) -> (25, 88)
  line L164 (25, 88) -> (7, 88)
  line L165 (7, 88) -> (7, 90)
  line L166 (7, 90) -> (25, 90)
  line L167 (25, 90) -> (25, 96)
  line L168 (25, 96) -> (7, 96)
  line L169 (7, 96) -> (7, 98)
  line L170 (7, 98) -> (25, 98)
  line L171 (25, 98) -> (25, 104)
  line L172 (25, 104) -> (7, 104)
  line L173 (7, 104) -> (7, 106)
  line L174 (7, 106) -> (25, 106)
  line L175 (25, 106) -> (25, 112)
  line L176 (25, 112) -> (7, 112)
  line L177 (7, 112) -> (7, 114)
  line L178 (7, 114) -> (25, 114)
  line L179 (25, 114) -> (25, 120)
  line L180 (25, 120) -> (7, 120)
  line L181 (7, 120) -> (7, 122)
  line L182 (7, 122) -> (25, 122)
  line L183 (25, 122) -> (25, 128)
  line L184 (25, 128) -> (7, 128)
  line L185 (7, 128) -> (7, 130)
  line L186 (7, 130) -> (25, 130)
  line L187 (25, 130) -> (25, 136)
  line L188 (25, 136) -> (7, 136)
  line L189 (7, 136) -> (7, 138)
  line L190 (7, 138) -> (25, 138)
  line L191 (25, 138) -> (25, 144)
  line L192 (25, 144) -> (7, 144)
  line L193 (7, 144) -> (7, 146)
  line L194 (7, 146) -> (25, 146)
  line L195 (25, 146) -> (25, 154)
  line L196 (25, 154) -> (7, 154)
  line L197 (7, 154) -> (7, 156)
  line L198 (7, 156) -> (25, 156)
  line L199 (25, 156) -> (25, 164)
  line L200 (23, 161) -> (23, 159)
  line L201 (23, 159) -> (-33, 159)
  line L202 (-33, 159) -> (-33, 161)
  line L203 (-33, 161) -> (23, 161)
  line L204 (4, 156) -> (4, 154)
  line L205 (4, 154) -> (-14, 154)
  line L206 (-14, 154) -> (-14, 156)
  line L207 (-14, 156) -> (4, 156)
  line L208 (23, 151) -> (23, 149)
  line L209 (23, 149) -> (-33, 149)
  line L210 (-33, 149) -> (-33, 151)
  line L211 (-33, 151) -> (23, 151)
  line L212 (23, 134) -> (23, 132)
  line L213 (23, 132) -> (-33, 132)
  line L214 (-33, 132) -> (-33, 134)
  line L215 (-33, 134) -> (23, 134)
  line L216 (23, 142) -> (23, 140)
  line L217 (23, 140) -> (-33, 140)
  line L218 (-33, 140) -> (-33, 142)
  line L219 (-33, 142) -> (23, 142)
  line L220 (23, 126) -> (23, 124)
  line L221 (23, 124) -> (-33, 124)
  line L222 (-33, 124) -> (-33, 126)
  line L223 (-33, 126) -> (23, 126)
  line L224 (4, 130) -> (4, 128)
  line L225 (4, 128) -> (-14, 128)
  line L226 (-14, 128) -> (-14, 130)
  line L227 (-14, 130) -> (4, 130)
  line L228 (4, 138) -> (4, 136)
  line L229 (4, 136) -> (-14, 136)
  line L230 (-14, 136) -> (-14, 138)
  line L231 (-14, 138) -> (4, 138)
  line L232 (4, 122) -> (4, 120)
  line L233 (4, 120) -> (-14, 120)
  line L234 (-14, 120) -> (-14, 122)
  line L235 (-14, 122) -> (4, 122)
  line L236 (23, 30) -> (23, 28)
  line L237 (23, 28) -> (-33, 28)
  line L238 (-33, 28) -> (-33, 30)
  line L239 (-33, 30) -> (23, 30)
  line L240 (23, 14) -> (23, 12)
  line L241 (23, 12) -> (-33, 12)
  line L242 (-33, 12) -> (-33, 14)
  line L243 (-33, 14) -> (23, 14)
  line L244 (23, -2) -> (23, -4)
  line L245 (23, -4) -> (-33, -4)
  line L246 (-33, -4) -> (-33, -2)
  line L247 (-33, -2) -> (23, -2)
  line L248 (23, 38) -> (23, 36)
  line L249 (23, 36) -> (-33, 36)
  line L250 (-33, 36) -> (-33, 38)
  line L251 (-33, 38) -> (23, 38)
  line L252 (4, 2) -> (4, 0)
  line L253 (4, 0) -> (-14, 0)
  line L254 (-14, 0) -> (-14, 2)
  line L255 (-14, 2) -> (4, 2)
  line L256 (4, 18) -> (4, 16)
  line L257 (4, 16) -> (-14, 16)
  line L258 (-14, 16) -> (-14, 18)
  line L259 (-14, 18) -> (4, 18)
  line L260 (4, 34) -> (4, 32)
  line L261 (4, 32) -> (-14, 32)
  line L262 (-14, 32) -> (-14, 34)
  line L263 (-14, 34) -> (4, 34)
  line L264 (4, 26) -> (4, 24)
  line L265 (4, 24) -> (-14, 24)
  line L266 (-14, 24) -> (-14, 26)
  line L267 (-14, 26) -> (4, 26)
  line L268 (4, 10) -> (4, 8)
  line L269 (4, 8) -> (-14, 8)
  line L270 (-14, 8) -> (-14, 10)
  line L271 (-14, 10) -> (4, 10)
  line L272 (4, -6) -> (4, -8)
  line L273 (4, -8) -> (-14, -8)
  line L274 (-14, -8) -> (-14, -6)
  line L275 (-14, -6) -> (4, -6)
  line L276 (4, -14) -> (4, -16)
  line L277 (4, -16) -> (-14, -16)
  line L278 (-14, -16) -> (-14, -14)
  line L279 (-14, -14) -> (4, -14)
  line L280 (23, -10) -> (23, -12)
  line L281 (23, -12) -> (-33, -12)
  line L282 (-33, -12) -> (-33, -10)
  line L283 (-33, -10) -> (23, -10)
  line L284 (23, 6) -> (23, 4)
  line L285 (23, 4) -> (-33, 4)
  line L286 (-33, 4) -> (-33, 6)
  line L287 (-33, 6) -> (23, 6)
  line L288 (23, 22) -> (23, 20)
  line L289 (23, 20) -> (-33, 20)
  line L290 (-33, 20) -> (-33, 22)
  line L291 (-33, 22) -> (23, 22)
  line L292 (4, -24) -> (-14, -24)
  line L293 (-14, -24) -> (-14, -22)
  line L294 (-14, -22) -> (4, -22)
  line L295 (4, -22) -> (4, -24)
  line L296 (23, -18) -> (23, -20)
  line L297 (23, -20) -> (-33, -20)
  line L298 (-33, -20) -> (-33, -18)
  line L299 (-33, -18) -> (23, -18)
  line L300 (4, 58) -> (4, 56)
  line L301 (4, 56) -> (-14, 56)
  line L302 (-14, 56) -> (-14, 58)
  line L303 (-14, 58) -> (4, 58)
  line L304 (23, 86) -> (23, 84)
  line L305 (23, 84) -> (-33, 84)
  line L306 (-33, 84) -> (-33, 86)
  line L307 (-33, 86) -> (23, 86)
  line L308 (23, 46.2715) -> (23, 44)
  line L309 (23, 44) -> (-33, 44)
  line L310 (-33, 44) -> (-33, 46.2715)
  line L311 (-33, 46.2715) -> (23, 46.2715)
  line L312 (4, 98) -> (4, 96)
  line L313 (4, 96) -> (-14, 96)
  line L314 (-14, 96) -> (-14, 98)
  line L315 (-14, 98) -> (4, 98)
  line L316 (4, 114) -> (4, 112)
  line L317 (4, 112) -> (-14, 112)
  line L318 (-14, 112) -> (-14, 114)
  line L319 (-14, 114) -> (4, 114)
  line L320 (23, 110) -> (23, 108)
  line L321 (23, 108) -> (-33, 108)
  line L322 (-33, 108) -> (-33, 110)
  line L323 (-33, 110) -> (23, 110)
  line L324 (23, 70) -> (23, 68)
  line L325 (23, 68) -> (-33, 68)
  line L326 (-33, 68) -> (-33, 70)
  line L327 (-33, 70) -> (23, 70)
  line L328 (4, 42) -> (4, 40)
  line L329 (4, 40) -> (-14, 40)
  line L330 (-14, 40) -> (-14, 42)
  line L331 (-14, 42) -> (4, 42)
  line L332 (4, 82) -> (4, 80)
  line L333 (4, 80) -> (-14, 80)
  line L334 (-14, 80) -> (-14, 82)
  line L335 (-14, 82) -> (4, 82)
  line L336 (-33, 116) -> (-33, 118)
  line L337 (-33, 118) -> (23, 118)
  line L338 (23, 118) -> (23, 116)
  line L339 (23, 116) -> (-33, 116)
  line L340 (23, 62) -> (23, 60)
  line L341 (23, 60) -> (-33, 60)
  line L342 (-33, 60) -> (-33, 62)
  line L343 (-33, 62) -> (23, 62)
  line L344 (4, 74) -> (4, 72)
  line L345 (4, 72) -> (-14, 72)
  line L346 (-14, 72) -> (-14, 74)
  line L347 (-14, 74) -> (4, 74)
  line L348 (4, 90) -> (4, 88)
  line L349 (4, 88) -> (-14, 88)
  line L350 (-14, 88) -> (-14, 90)
  line L351 (-14, 90) -> (4, 90)
  line L352 (4, 50) -> (4, 48)
  line L353 (4, 48) -> (-14, 48)
  line L354 (-14, 48) -> (-14, 50)
  line L355 (-14, 50) -> (4, 50)
  line L356 (23, 102) -> (23, 100)
  line L357 (23, 100) -> (-32.9874, 100)
  line L358 (-32.9874, 100) -> (-32.9874, 102)
  line L359 (-32.9874, 102) -> (23, 102)
  line L360 (4, 106) -> (4, 104)
  line L361 (4, 104) -> (-14, 104)
  line L362 (-14, 104) -> (-14, 106)
  line L363 (-14, 106) -> (4, 106)
  line L364 (4, 66) -> (4, 64)
  line L365 (4, 64) -> (-14, 64)
  line L366 (-14, 64) -> (-14, 66)
  line L367 (-14, 66) -> (4, 66)
  line L368 (23, 54) -> (23, 52)
  line L369 (23, 52) -> (-33, 52)
  line L370 (-33, 52) -> (-33, 54)
  line L371 (-33, 54) -> (23, 54)
  line L372 (-33, 94) -> (23, 94)
  line L373 (23, 94) -> (23, 92)
  line L374 (23, 92) -> (-33, 92)
  line L375 (-33, 92) -> (-33, 94)
  line L376 (23, 78) -> (23, 76)
  line L377 (23, 76) -> (-33, 76)
  line L378 (-33, 76) -> (-33, 78)
  line L379 (-33, 78) -> (23, 78)
  line L380 (4, 146) -> (4, 144)
  line L381 (4, 144) -> (-14, 144)
  line L382 (-14, 144) -> (-14, 146)
  line L383 (-14, 146) -> (4, 146)
  line L384 (4, -32) -> (4, -34)
  line L385 (4, -34) -> (-14, -34)
  line L386 (-14, -34) -> (-14, -32)
  line L387 (-14, -32) -> (4, -32)
  line L388 (23, -29) -> (-33, -29)
  line L389 (-33, -29) -> (-33, -27)
  line L390 (-33, -27) -> (23, -27)
  line L391 (23, -27) -> (23, -29)
  line L392 (35, -80) -> (35, 164)
  line L393 (-40.5, -42) -> (-40.5, 164)
  constraint perpendicular L390 L392
  constraint perpendicular L0 L393
extrude "Extrude41" cut 5 faces at (-13, -164, 3.3333) (-5, -164, 1.6667) (2, -164, 1.6667) (16, -164, 1.6667) (29, -164, 3.3333) along direction (0, 1, 0) blind 68
extrude "Extrude42" add 1 faces at (-6.6667, 80, 10.3333) along direction (0, -1, 0) blind 6
